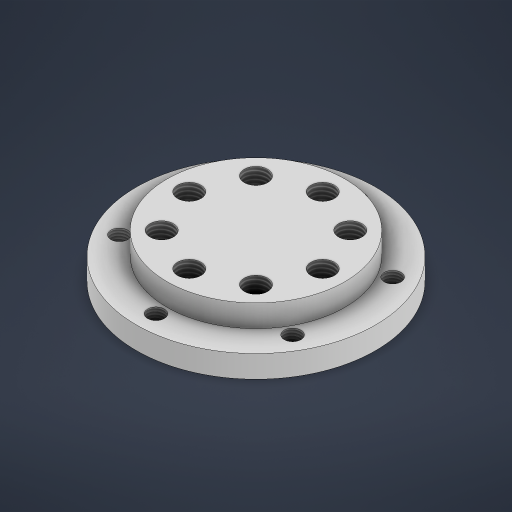
# Autodesk Inventor part: OutPutPlate
Saved by Autodesk Inventor 2024 (Build 280153000, 153)
## iProperties
Created: 2024-01-31
Part Number: OutPutPlate
Material: Generic
Document SubType Name: Modeling
Designer: avsar
Density: 1 g/cm^3
Appearance: Default
Author: avsar
Autodesk Inventor part; units mm, degrees
ref_plane "YZ Plane" through (0, 0, 0) normal (1, 0, 0) x (0, 1, 0)
ref_plane "XZ Plane" through (0, 0, 0) normal (0, 1, 0) x (-1, 0, 0)
ref_plane "XY Plane" through (0, 0, 0) normal (0, 0, 1) x (1, 0, 0)
sketch "Sketch1" plane through (0, 0, 0) normal (0, 1, 0) x (-1, 0, 0)
  circle A0 centre (0, 0) radius 21.5
  circle A1 centre (0, -18) radius 1.5
  circle A2 centre (15.5885, -9) radius 1.5
  circle A3 centre (15.5885, 9) radius 1.5
  circle A4 centre (0, 18) radius 1.5
  circle A5 centre (-15.5885, 9) radius 1.5
  circle A6 centre (-15.5885, -9) radius 1.5
  dimension "d0" = 43
  dimension "d1" = 3
  dimension "d2" = 18
  dimension "d5" = 360
  constraints: 7 centre point, 1 coincident, 1 vertical alignment, 13 other
  measures "d0" diameter of A0
  measures "d1" diameter of A1
  measures "d2" distance of point (0, 0) A1.centre
extrude "Extrusion1" add sketch "Sketch1" along normal blind 4
sketch "Sketch2" plane through (0, 4, 0) normal (0, 1, 0) x (1, 0, 0)
  circle A0 centre (0, 0) radius 16
  dimension "d9" = 32
  constraints: 1 centre point, 1 coincident
  measures "d9" diameter of A0
extrude "Extrusion2" add sketch "Sketch2" along normal blind 4
sketch "Sketch3" plane through (0, 8, 0) normal (0, 1, 0) x (1, 0, 0)
  circle A0 centre (0, 12) radius 2.1
  circle A1 centre (-8.4853, 8.4853) radius 2.1
  circle A2 centre (-12, 0) radius 2.1
  circle A3 centre (-8.4853, -8.4853) radius 2.1
  circle A4 centre (0, -12) radius 2.1
  circle A5 centre (8.4853, -8.4853) radius 2.1
  circle A6 centre (12, 0) radius 2.1
  circle A7 centre (8.4853, 8.4853) radius 2.1
  point P0 (0, 0)
  dimension "d27" = 4.2
  dimension "d32" = 360
  dimension "d44" = 12
  constraints: 8 centre point, 1 vertical alignment, 17 other
  measures "d27" diameter of A0
  measures "d44" distance of point (0, 0) A0.centre
extrude "Extrusion3" cut sketch "Sketch3" against normal blind 4
thread "Thread7" size "M4x0.7" class "6H" standard "ANSI Metric M Profile" full length
thread "Thread8" size "M4x0.7" class "6H" standard "ANSI Metric M Profile" full length
thread "Thread9" size "M4x0.7" class "6H" standard "ANSI Metric M Profile" full length
thread "Thread10" size "M4x0.7" class "6H" standard "ANSI Metric M Profile" full length
thread "Thread11" size "M4x0.7" class "6H" standard "ANSI Metric M Profile" full length
thread "Thread12" size "M4x0.7" class "6H" standard "ANSI Metric M Profile" full length
thread "Thread13" size "M4x0.7" class "6H" standard "ANSI Metric M Profile" full length
thread "Thread14" size "M4x0.7" class "6H" standard "ANSI Metric M Profile" full length
thread "Thread15" size "M3x0.5" class "6H" standard "ANSI Metric M Profile" full length
thread "Thread16" size "M3x0.5" class "6H" standard "ANSI Metric M Profile" full length
thread "Thread17" size "M3x0.5" class "6H" standard "ANSI Metric M Profile" full length
thread "Thread18" size "M3x0.5" class "6H" standard "ANSI Metric M Profile" full length
thread "Thread19" size "M3x0.5" class "6H" standard "ANSI Metric M Profile" full length
thread "Thread20" size "M3x0.5" class "6H" standard "ANSI Metric M Profile" full length
sketch "Sketch4" plane through (0, 0, 0) normal (0, -1, 0) x (1, 0, 0)
  circle A0 centre (0, 0) radius 6
  dimension "d65" = 12
  constraints: 1 centre point, 1 coincident
  measures "d65" diameter of A0
extrude "Extrusion4" cut sketch "Sketch4" against normal blind 5
body "Solid1"
